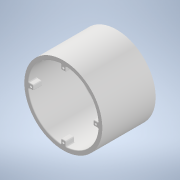
# Autodesk Inventor part: Marshmallow
Saved by Autodesk Inventor 2020 (Build 240168000, 168)
## iProperties
Created: 2020-08-08
Part Number: Marshmallow
Material: Generic
Document SubType Name: Modeling
Designer: reide
Density: 1 g/cm^3
Appearance: Default
Author: reide
Autodesk Inventor part; units mm, degrees
ref_plane "YZ Plane" through (0, 0, 0) normal (1, 0, 0) x (0, 1, 0)
ref_plane "XZ Plane" through (0, 0, 0) normal (0, 1, 0) x (-1, 0, 0)
ref_plane "XY Plane" through (0, 0, 0) normal (0, 0, 1) x (1, 0, 0)
sketch "Sketch2" plane through (0, 0, 0) normal (0, 0, 1) x (1, 0, 0)
  line L0 (0, 0) -> (0, -80)
  line L1 (0, -80) -> (0, -53)
  circle A0 centre (0, -53) radius 12.5
  line L2 (0, -80) -> (0, -42.5)
  circle A1 centre (0, -42.5) radius 47.5
  line L3 (0, -53) -> (0, -13)
  circle A2 centre (0, -13) radius 6.4
  dimension "d1" = 27
  dimension "d2" = 25
  dimension "d3" = 37.5
  dimension "d4" = 95
  dimension "d5" = 40
  dimension "d6" = 12.8
  constraints: 8 end point, 3 centre point, 3 coincident, 3 point on line, 1 vertical
  measures "d1" distance of L0.end L1.end
  measures "d2" diameter of A0
  measures "d3" distance of L0.end L2.end
  measures "d4" diameter of A1
  measures "d5" distance of L3.start L3.end
  measures "d6" diameter of A2
extrude "Extrusion1" add sketch "Sketch2" along normal blind 5
sketch "Sketch3" plane through (0, -42.5, 5) normal (0, 0, 1) x (1, 0, 0)
  circle A0 centre (0, 0) radius 47.5 projected
  circle A1 centre (0, 29.5) radius 6.4 projected
  circle A2 centre (0, -10.5) radius 12.5 projected
  circle A3 centre (0, 0) radius 42.5
  point P0 (0, 42.5)
  dimension "d9" = 85
  constraints: 1 centre point, 1 coincident
  measures "d9" diameter of A3
extrude "Extrusion2" add sketch "Sketch3" along normal blind 60 contours A0
sketch "Sketch4" plane through (0, -42.5, 65) normal (0, 0, 1) x (1, 0, 0)
  circle A0 centre (0, 0) radius 47.5 projected
  circle A1 centre (0, 0) radius 42.5 projected
  circle A2 centre (0, 0) radius 42.5 projected
  line L0 (0, -42.5) -> (0, -36.5)
  line L1 (0, -36.5) -> (-3, -36.5)
  line L2 (-3, -36.5) -> (3, -36.5)
  line L3 (-3, -36.5) -> (3, -36.5)
  line L4 (3, -36.5) -> (3, -42.5)
  line L5 (3, -42.5) -> (-3, -42.5)
  line L6 (-3, -42.5) -> (-3, -36.5)
  line L7 (0, 0) -> (-25.8921, 0)
  circle A3 centre (0, -39.5) radius 1.25
  line L8 (42.5, 0) -> (36.5, 0)
  line L9 (36.5, 0) -> (36.5, -3)
  line L10 (36.5, -3) -> (36.5, 3)
  line L11 (36.5, -3) -> (36.5, 3)
  line L12 (36.5, 3) -> (42.5, 3)
  line L13 (42.5, 3) -> (42.5, -3)
  line L14 (42.5, -3) -> (36.5, -3)
  circle A4 centre (39.5, 0) radius 1.25
  line L15 (0, 42.5) -> (0, 36.5)
  line L16 (0, 36.5) -> (3, 36.5)
  line L17 (3, 36.5) -> (-3, 36.5)
  line L18 (3, 36.5) -> (-3, 36.5)
  line L19 (-3, 36.5) -> (-3, 42.5)
  line L20 (-3, 42.5) -> (3, 42.5)
  line L21 (3, 42.5) -> (3, 36.5)
  circle A5 centre (0, 39.5) radius 1.25
  line L22 (-42.5, 0) -> (-36.5, 0)
  line L23 (-36.5, 0) -> (-36.5, 3)
  line L24 (-36.5, 3) -> (-36.5, -3)
  line L25 (-36.5, 3) -> (-36.5, -3)
  line L26 (-36.5, -3) -> (-42.5, -3)
  line L27 (-42.5, -3) -> (-42.5, 3)
  line L28 (-42.5, 3) -> (-36.5, 3)
  circle A6 centre (-39.5, 0) radius 1.25
  point P0 (0, 42.5)
  point P1 (-3, 42.394)
  point P2 (3, 42.394)
  point P3 (42.394, 3)
  point P4 (36.5, 3)
  point P5 (36.5, 0)
  point P6 (42.394, -3)
  point P7 (3, -42.394)
  point P8 (-3, -42.394)
  point P9 (-36.5, 0)
  point P10 (-42.394, 3)
  point P11 (-42.394, -3)
  point P12 (-36.5, -3)
  dimension "d12" = 6
  dimension "d13" = 3
  dimension "d14" = 6
  dimension "d15" = 2.5
  dimension "d18" = 360
  constraints: 58 end point, 4 centre point, 4 point on line, 2 horizontal, 2 parallel, 2 perpendicular, 1 midpoint, 1 point on circle, 1 vertical, 65 other
  measures "d12" distance of L0.start L0.end
  measures "d13" distance of L0.end L1.end
  measures "d14" distance of L1.end L2.end
  measures "d15" diameter of A3
extrude "Extrusion3" add sketch "Sketch4" against normal blind 10 contours L8 A4 L10 L12 A1 | A1 L14 L9 L8 A4 | L21 L16 L15 A5 A1 | A1 L0 A3 L2 L4 | L15 A5 L17 L19 A1 | A1 L6 L1 L0 A3 | L28 L23 L22 A6 A1 | A1 L22 A6 L24 L26
fillet "Fillet1" radius 1 16 edges at (-3, -6, 60) (3, -6, 60) (36.5, -39.5, 60) (36.5, -45.5, 60) (-36.5, -39.5, 60) (-36.5, -45.5, 60) (3, -0.106, 60) (-3, -0.106, 60) (-42.394, -39.5, 60) (-42.394, -45.5, 60) (3, -79, 60) (-3, -79, 60) (42.394, -45.5, 60) (42.394, -39.5, 60) (-3, -84.894, 60) (3, -84.894, 60)
fillet "Fillet2" radius 1 32 edges at (42.0472, -39.1722, 65) (39.4034, -39.5, 65) (36.7929, -39.7929, 65) (36.5, -42.5, 65) (36.7929, -45.2071, 65) (39.4034, -45.5, 65) (42.0472, -45.8278, 65) (30.052, -72.552, 65) (3.3278, -84.5472, 65) (3, -81.9034, 65) (2.7071, -79.2929, 65) (0, -79, 65) (-2.7071, -79.2929, 65) (-3, -81.9034, 65) (-3.3278, -84.5472, 65) (-30.052, -72.552, 65) (-42.0472, -45.8278, 65) (-39.4034, -45.5, 65) (-36.7929, -45.2071, 65) (-36.5, -42.5, 65) (-36.7929, -39.7929, 65) (-39.4034, -39.5, 65) (-42.0472, -39.1722, 65) (-30.052, -12.448, 65) (-3.3278, -0.4528, 65) (-3, -3.0966, 65) (-2.7071, -5.7071, 65) (0, -6, 65) (2.7071, -5.7071, 65) (3, -3.0966, 65) (3.3278, -0.4528, 65) (30.052, -12.448, 65)
fillet "Fillet3" radius 1 4 edges at (-12.5, -53, 5) (-6.4, -13, 5) (-12.5, -53, 0) (-6.4, -13, 0)
fillet "Fillet4" radius 1 1 edges at (-42.5, -42.5, 5)
sketch "Sketch5" plane through (0, -42.5, 0) normal (0, 0, -1) x (-1, 0, 0)
  point P0 (0, 42.5)
sketch "Sketch6" plane through (0, -42.5, 0) normal (0, 0, -1) x (-1, 0, 0)
  circle A0 centre (18.7437, -10.9845) radius 1.7 projected
  circle A1 centre (-18.7437, -10.0155) radius 1.7 projected
  circle A2 centre (18.7437, -10.9845) radius 2
  circle A3 centre (-18.7437, -10.0155) radius 2
  point P0 (0, 42.5)
  dimension "d26" = 4
  dimension "d27" = 4
  constraints: 2 centre point, 2 coincident
  measures "d26" diameter of A2
  measures "d27" diameter of A3
extrude "Extrusion4" cut sketch "Sketch6" against normal blind 5 contours A0 | A1 | A2 | A3
fillet "Fillet5" radius 1 4 edges at (-16.7437, -53.4845, 5) (-16.7437, -53.4845, 0) (20.7437, -52.5155, 0) (20.7437, -52.5155, 5)
body "Solid1"
